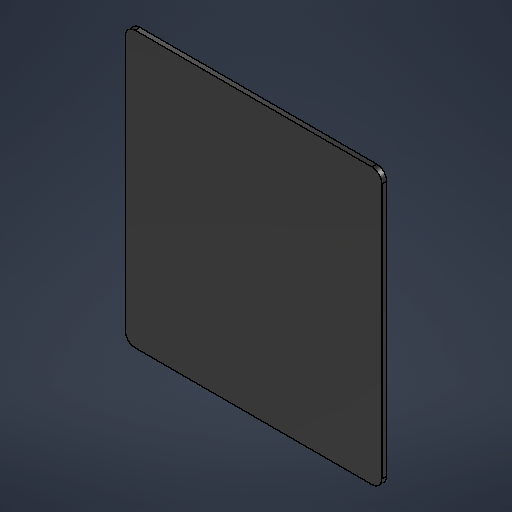
# Autodesk Inventor part: Inner Side Panel
Saved by Autodesk Inventor 2026 (Build 300175050, 175E)
## iProperties
Created: 2025-05-20
Part Number: Inner Side Panel
Material: PC/ABS Plastic
Document SubType Name: Modeling
Designer: Joshua Eah
Density: 1.1 g/cm^3
Appearance: Smooth - White
Author: Joshua Eah
Autodesk Inventor part; units mm, degrees
ref_plane "YZ Plane" through (0, 0, 0) normal (1, 0, 0) x (0, 1, 0)
ref_plane "XZ Plane" through (0, 0, 0) normal (0, 1, 0) x (-1, 0, 0)
ref_plane "XY Plane" through (0, 0, 0) normal (0, 0, 1) x (1, 0, 0)
sketch "Sketch1" plane through (0, 0, 0) normal (0, 0, 1) x (1, 0, 0)
  line L0 (0, 0) -> (167, 0)
  line L1 (167, 0) -> (167, 179)
  line L2 (167, 179) -> (0, 179)
  line L3 (0, 179) -> (0, 0)
  dimension "d0" = 179
  dimension "d1" = 167
  constraints: 8 end point, 2 parallel, 1 horizontal, 1 perpendicular
  measures "d0" distance of L1.end L0.end
  measures "d1" distance of L0.start L0.end
extrude "Extrusion1" add sketch "Sketch1" along normal blind 3.175
fillet "Fillet1" radius 6.35 4 edges at (167, 179, 1.5875) (0, 179, 1.5875) (167, 0, 1.5875) (0, 0, 1.5875)
body "Solid1"
